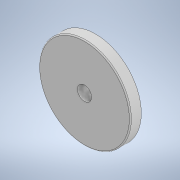
# Autodesk Inventor part: parafuso da polia
Saved by Autodesk Inventor 2022.1 (Build 261234020, 234B)
## iProperties
Created: 2023-08-25
Part Number: parafuso da polia
Material: Generic
Document SubType Name: Modeling
Designer: SENAI
Density: 1 g/cm^3
Appearance: Default
Author: SENAI
Autodesk Inventor part; units mm, degrees
ref_plane "YZ Plane" through (0, 0, 0) normal (1, 0, 0) x (0, 1, 0)
ref_plane "XZ Plane" through (0, 0, 0) normal (0, 1, 0) x (-1, 0, 0)
ref_plane "XY Plane" through (0, 0, 0) normal (0, 0, 1) x (1, 0, 0)
sketch "Sketch1" plane through (0, 0, 0) normal (0, 0, 1) x (1, 0, 0)
  circle A0 centre (0, 0) radius 22.5
  circle A1 centre (0, 0) radius 3.5
  dimension "d0" = 45
  dimension "d1" = 7
  constraints: 2 centre point, 2 coincident
  measures "d0" diameter of A0
  measures "d1" diameter of A1
extrude "Extrusion1" add sketch "Sketch1" along normal blind 5.4
fillet "Fillet1" radius 0.5 1 edges at (-22.5, 0, 5.4)
body "Solid1"
